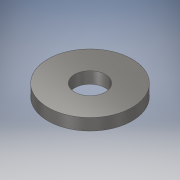
# Autodesk Inventor part: ワッシャー_M8＿3.2mm
Saved by Autodesk Inventor 2019 (Build 230136000, 136)
## iProperties
Created: 2020-10-19
Part Number: ワッシャー_M8＿3.2mm
Material: ステンレス鋼
Document SubType Name: Modeling
Designer: zhept
Density: 8 g/cm^3
Appearance: 半つや出し
Author: zhept
Autodesk Inventor part; units mm, degrees
ref_plane "YZ Plane" through (0, 0, 0) normal (1, 0, 0) x (0, 1, 0)
ref_plane "XZ Plane" through (0, 0, 0) normal (0, 1, 0) x (-1, 0, 0)
ref_plane "XY Plane" through (0, 0, 0) normal (0, 0, 1) x (1, 0, 0)
sketch "スケッチ1" plane through (0, 0, 0) normal (0, 1, 0) x (-1, 0, 0)
  circle A0 centre (0, 0) radius 4.2
  circle A1 centre (0, 0) radius 11.5
  dimension "d0" = 8.4
  dimension "d1" = 23
  constraints: 2 centre point, 2 coincident
  measures "d0" diameter of A0
  measures "d1" diameter of A1
extrude "押し出し1" add sketch "スケッチ1" along normal blind 3.2
